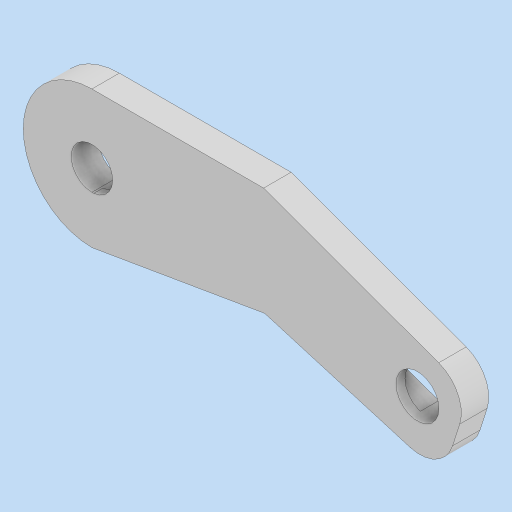
# Autodesk Inventor part: pata_superior_v3
Saved by Autodesk Inventor 2024 (Build 280153000, 153)
## iProperties
Created: 2024-07-27
Part Number: pata_superior_v3
Material: Generic
Document SubType Name: Modeling
Designer: MxMon
Density: 1 g/cm^3
Appearance: Default
Author: MxMon
Autodesk Inventor part; units mm, degrees
ref_plane "YZ Plane" through (0, 0, 0) normal (1, 0, 0) x (0, 1, 0)
ref_plane "XZ Plane" through (0, 0, 0) normal (0, 1, 0) x (-1, 0, 0)
ref_plane "XY Plane" through (0, 0, 0) normal (0, 0, 1) x (1, 0, 0)
sketch "Sketch1" plane through (0, 0, 0) normal (0, 0, 1) x (1, 0, 0)
  arc A0 (0.2884, 3.0112) -> (0.2884, -3.0112) centre (0, 0) ccw
  arc A1 (15.7, -2.275) -> (15.7, 2.275) centre (15.7, 0) ccw
  line L0 (0, 3.025) -> (15.7, 2.275)
  line L1 (0, -3.025) -> (15.7, -2.275)
  dimension "d0" = 6.05
  dimension "d2" = 15.7
  dimension "d3" = 4.55
  constraints: 6 point on circle, 4 end point, 4 vertical alignment, 2 centre point, 2 point on line, 1 coincident, 1 horizontal alignment
  measures "d0" diameter of A0
  measures "d2" distance of A1.centre point (0, 0)
  measures "d3" distance of L1.end L0.end
sketch "Sketch15" plane through (0, 0, 0) normal (0, 0, 1) x (1, 0, 0)
  arc A0 (0, 10) -> (0, -10) centre (0, 0) ccw
  line L0 (0, 10) -> (25, 10)
  line L1 (0, -10) -> (25.1576, -5.7133)
  line L2 (25, 10) -> (55, -0.9191)
  line L3 (25.1576, -5.7133) -> (51.033, -13.4271)
  line L4 (55, -0.9191) -> (51.033, -13.4271)
  dimension "d92" = 20
  dimension "d93" = 25
  dimension "d94" = 160
  dimension "d96" = 13.122
  dimension "d97" = 153.73
  dimension "d99" = 9.67
  dimension "d100" = 30
  dimension "d102" = 51.033
  constraints: 10 end point, 2 point on circle, 2 vertical alignment, 1 centre point, 1 coincident, 1 tangent
  measures "d92" diameter of A0
  measures "d93" distance of L0.start L0.end
  measures "d94" angle of L0 L2
  measures "d96" distance of L3.end L2.end
  measures "d97" angle of L1 L3
  measures "d99" angle of L1 L0
  measures "d100" horizontal distance of L2.end L0.end
  measures "d102" horizontal distance of L3.end L1.start
extrude "Extrusion15" add sketch "Sketch15" along normal blind 4
extrude "Extrusion16" cut sketch "Sketch1" along normal blind 2.7 contours L0 A1 L1 A0
sketch "Sketch16" plane through (0, 0, 0) normal (0, 0, -1) x (-1, 0, 0)
  line L0 (-51.033, -13.4271) -> (-55, -0.9191) construction
  line L1 (-53.1492, -6.7546) -> (-25.1636, 1.5882) construction
  line L2 (-25.1576, -5.7133) -> (-51.033, -13.4271) construction
  arc A0 (-47.9716, -1.9693) -> (-46.1965, -7.9238) centre (-47.4074, -5.0429) ccw
  arc A1 (-31.7118, -2.7378) -> (-33.0116, 1.6226) centre (-32.3617, -0.5576) ccw
  line L3 (-48.3001, -2.0482) -> (-33.0116, 1.6226)
  line L4 (-46.5146, -8.0377) -> (-31.7118, -2.7378)
  point P0 (0, 0)
  point P1 (-53.0165, -7.1731)
  point P2 (-46.5146, -8.0377)
  dimension "d107" = 6.25
  dimension "d108" = 6
  dimension "d109" = 4.55
  dimension "d110" = 15.7
  dimension "d111" = 3.125
  dimension "d112" = 2.275
  dimension "d113" = 7
  constraints: 6 end point, 5 point on circle, 5 point on line, 2 centre point, 2 symmetric about line, 1 midpoint, 1 parallel
  measures "d107" diameter of A0
  measures "d108" distance of point (-53.017, -7.173) A0.centre
  measures "d109" diameter of A1
  measures "d110" distance of A1.centre A0.centre
  measures "d111" distance from line of L1 L3.start
  measures "d112" distance from line of L1 L3.end
  measures "d113" distance of L0.start L1.start
extrude "Extrusion17" cut sketch "Sketch16" against normal blind 2.7 contours L3 A1 L4 A0
sketch "Sketch17" plane through (0, 0, 2.7) normal (0, 0, -1) x (-1, 0, 0)
  arc A0 (0, -10) -> (0, 10) centre (0, 0) ccw projected
  line L0 (0, -3.025) -> (-15.7, -2.275) projected
  circle A1 centre (0, 0) radius 3.025
  arc A2 (-48.3001, -2.0482) -> (-46.5146, -8.0377) centre (-47.4074, -5.0429) ccw projected
  circle A3 centre (-47.4074, -5.0429) radius 3.125
  point P0 (-0.2884, -3.0112)
  point P1 (-48.3001, -2.0482)
  constraints: 2 coincident, 6 other
extrude "Extrusion18" cut sketch "Sketch17" against normal through all
fillet "Fillet5" radius 5 2 edges at (55, -0.9191, 2) (51.033, -13.4271, 2)
body "Solid3"
